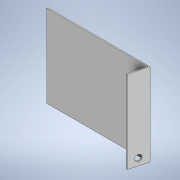
# Autodesk Inventor part: bottomCover
Saved by Autodesk Inventor 2020.3 (Build 243373000, 373)
## iProperties
Created: 2021-03-06
Part Number: bottomCover
Material: Generic
Document SubType Name: Modeling
Designer: allofus
Density: 1 g/cm^3
Appearance: Default
Author: allofus
Autodesk Inventor part; units mm, degrees
ref_plane "YZ Plane" through (0, 0, 0) normal (1, 0, 0) x (0, 1, 0)
ref_plane "XZ Plane" through (0, 0, 0) normal (0, 1, 0) x (-1, 0, 0)
ref_plane "XY Plane" through (0, 0, 0) normal (0, 0, 1) x (1, 0, 0)
sketch "Sketch1" plane through (0, 0, 0) normal (0, 1, 0) x (-1, 0, 0)
  line L0 (0, 0) -> (5, 0)
  line L1 (5, 161) -> (0, 161)
  line L2 (0, 0) -> (197.574, 0)
  line L3 (197.574, 0) -> (197.574, 2)
  line L4 (197.574, 2) -> (0, 2)
  line L5 (0, 2) -> (0, 0)
  line L6 (0, 2) -> (8.9293, 35.3244)
  line L7 (0, 2) -> (34.5, 2) construction
  line L8 (8.9293, 35.3244) -> (6.9974, 35.8421)
  line L9 (6.9974, 35.8421) -> (-2.6065, 0)
  line L10 (-2.6065, 0) -> (0, 0)
  line L11 (8.9293, 35.3244) -> (6.8587, 35.3244)
  line L12 (197.574, 2) -> (197.0381, 0)
  line L13 (197.574, 2) -> (199.6446, 2) construction
  dimension "d1" = 5
  dimension "d2" = 197.574
  dimension "d3" = 2
  dimension "d4" = 34.5
  dimension "d5" = 75
  dimension "d6" = 2
  dimension "d11" = 105
  constraints: 28 end point, 5 horizontal, 3 parallel, 3 perpendicular, 2 equal length, 2 point on line, 1 collinear
  measures "d1" distance of L1.start L1.end
  measures "d2" distance of L4.end L3.end
  measures "d3" distance of L3.end L2.end
  measures "d4" distance of L4.end L6.end
  measures "d5" angle of L7 L6
  measures "d6" distance of L6.end L8.end
  measures "d11" angle of L12 L13
extrude "Extrusion1" add sketch "Sketch1" along normal blind 161 contours L5 L4 L12 L2 L0 | L10 L9 L11 L6 L5
sketch "Sketch3" plane through (-8.9293, 0, 35.3244) normal (-0.9659258, 0, -0.258819) x (-0.258819, 0, 0.9659258)
  circle A0 centre (-17.9972, 13.5211) radius 6
  line L0 (-19.9848, 8.9507) -> (-15.1606, 8.9507)
  line L1 (-15.1606, 8.9507) -> (-15.1606, -1.5715)
  line L2 (-15.1606, -1.5715) -> (-19.9848, -1.5715)
  line L3 (-19.9848, -1.5715) -> (-19.9848, 8.9507)
  point P0 (-36.4319, 0)
  point P1 (-15.1606, 8.234)
  point P2 (-19.9848, 7.8599)
  dimension "d12" = 12
  constraints: 8 end point, 2 parallel, 1 centre point, 1 horizontal, 1 perpendicular
  measures "d12" diameter of A0
extrude "Extrusion3" cut sketch "Sketch3" against normal blind 58.2625 contours A0 L1 L0 L3 | L3 L0 L1 A0
body "Solid1"
